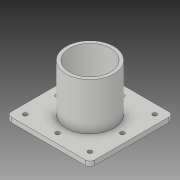
# Autodesk Inventor part: duct_mount
Saved by Autodesk Inventor 2019 (Build 230136000, 136)
## iProperties
Created: 2020-07-02
Part Number: duct_mount
Material: Generic
Document SubType Name: Modeling
Designer: devon
Density: 1 g/cm^3
Appearance: Default
Author: devon
Autodesk Inventor part; units mm, degrees
ref_plane "YZ Plane" through (0, 0, 0) normal (1, 0, 0) x (0, 1, 0)
ref_plane "XZ Plane" through (0, 0, 0) normal (0, 1, 0) x (-1, 0, 0)
ref_plane "XY Plane" through (0, 0, 0) normal (0, 0, 1) x (1, 0, 0)
sketch "Sketch1" plane through (0, 0, 0) normal (0, 1, 0) x (-1, 0, 0)
  line L0 (44.45, 44.45) -> (-44.45, 44.45)
  line L1 (-44.45, 44.45) -> (-44.45, -44.45)
  line L2 (-44.45, -44.45) -> (44.45, -44.45)
  line L3 (44.45, -44.45) -> (44.45, 44.45)
  line L4 (44.45, 44.45) -> (-44.45, -44.45) construction
  line L5 (-44.45, 44.45) -> (44.45, -44.45) construction
  point P0 (0, 0)
  dimension "d0" = 88.9
  dimension "d1" = 88.9
  constraints: 12 end point, 2 midpoint, 2 parallel, 1 horizontal, 1 perpendicular
  measures "d0" distance of L1.end L2.end
  measures "d1" distance of L2.end L0.start
extrude "Extrusion1" add sketch "Sketch1" along normal blind 5
sketch "Sketch2" plane through (0, 5, 0) normal (0, 1, 0) x (1, 0, 0)
  circle A0 centre (0, 0) radius 25.4
  dimension "d4" = 50.8
  constraints: 1 centre point, 1 coincident
  measures "d4" diameter of A0
extrude "Extrusion2" add sketch "Sketch2" along normal blind 50
sketch "Sketch3" plane through (0, 5, 0) normal (0, 1, 0) x (1, 0, 0)
  line L0 (44.45, 44.45) -> (-44.45, 44.45) projected
  line L1 (-44.45, 44.45) -> (-44.45, -44.45) projected
  line L2 (44.45, -44.45) -> (44.45, 44.45) projected
  line L3 (-44.45, -44.45) -> (44.45, -44.45) projected
  point P0 (0, 0)
  point P1 (-34.45, 34.45)
  point P2 (0, 34.45)
  point P3 (34.45, 34.45)
  point P4 (34.45, 0)
  point P5 (34.45, -34.45)
  point P6 (0, -34.45)
  point P7 (-34.45, -34.45)
  point P8 (-34.45, 0)
  dimension "d14" = 10
  dimension "d15" = 10
  dimension "d16" = 10
  dimension "d17" = 0
  dimension "d18" = 10
  dimension "d19" = 10
  dimension "d20" = 10
  dimension "d21" = 0
  dimension "d22" = 10
  dimension "d23" = 10
  dimension "d24" = 10
  dimension "d25" = 0
  dimension "d26" = 10
  dimension "d27" = 10
  dimension "d28" = 10
  dimension "d29" = 0
  measures "d14" distance from line of L0 point (-34.45, 34.45)
  measures "d15" distance from line of L1 point (-34.45, 34.45)
  measures "d16" distance from line of L0 point (0, 34.45)
  measures "d17" horizontal distance of point (0, 0) point (0, 34.45)
  measures "d18" distance from line of L0 point (34.45, 34.45)
  measures "d19" distance from line of L2 point (34.45, 34.45)
  measures "d20" distance from line of L2 point (34.45, 0)
  measures "d21" vertical distance of point (0, 0) point (34.45, 0)
  measures "d22" distance from line of L2 point (34.45, -34.45)
  measures "d23" distance from line of L3 point (34.45, -34.45)
  measures "d24" distance from line of L3 point (0, -34.45)
  measures "d25" horizontal distance of point (0, 0) point (0, -34.45)
  measures "d26" distance from line of L3 point (-34.45, -34.45)
  measures "d27" distance from line of L1 point (-34.45, -34.45)
  measures "d28" distance from line of L1 point (-34.45, 0)
  measures "d29" vertical distance of point (0, 0) point (-34.45, 0)
hole "Hole1" at (-34.45, 5, -34.45) at (0, 5, -34.45) at (34.45, 5, -34.45) at (34.45, 5, 0) at (34.45, 5, 34.45) at (0, 5, 34.45) at (-34.45, 5, 34.45) at (-34.45, 5, 0) direction (0, -1, 0) diameter 4.496 end through all clearance for "Socket Head Cap Screw" size "#8" standard "Ansi Unified Screw Threads"
sketch "Sketch4" plane through (0, 55, 0) normal (0, 1, 0) x (1, 0, 0)
  circle A0 centre (0, 0) radius 21.9
  dimension "d30" = 43.8
  constraints: 1 centre point, 1 coincident
  measures "d30" diameter of A0
extrude "Extrusion3" cut sketch "Sketch4" against normal up to next
fillet "Fillet1" radius 5 4 edges at (-44.45, 2.5, 44.45) (44.45, 2.5, 44.45) (44.45, 2.5, -44.45) (-44.45, 2.5, -44.45)
body "Solid1"
